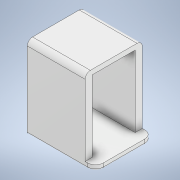
# Autodesk Inventor part: Fridge-Body
Saved by Autodesk Inventor 2020 (Build 240168000, 168)
## iProperties
Created: 2020-02-06
Part Number: Fridge-Body
Material: Generic
Document SubType Name: Modeling
Designer: Simon
Density: 1 g/cm^3
Appearance: Smooth - White
Author: Simon
Autodesk Inventor part; units mm, degrees
ref_plane "YZ Plane" through (0, 0, 0) normal (1, 0, 0) x (0, 1, 0)
ref_plane "XZ Plane" through (0, 0, 0) normal (0, 1, 0) x (-1, 0, 0)
ref_plane "XY Plane" through (0, 0, 0) normal (0, 0, 1) x (1, 0, 0)
sketch "Sketch1" plane through (0, 0, 0) normal (1, 0, 0) x (0, 1, 0)
  line L0 (0, 139.7) -> (396.875, 139.7)
  line L1 (396.875, 139.7) -> (396.875, -139.7)
  line L2 (396.875, -139.7) -> (0, -139.7)
  line L3 (0, -139.7) -> (0, 139.7)
  line L4 (396.875, -139.7) -> (0, 139.7) construction
  line L5 (23.8125, -104.775) -> (373.0625, -104.775)
  line L6 (373.0625, -104.775) -> (373.0625, 104.775)
  line L7 (373.0625, 104.775) -> (23.8125, 104.775)
  line L8 (23.8125, 104.775) -> (23.8125, -104.775)
  line L9 (23.8125, -104.775) -> (373.0625, 104.775) construction
  line L10 (373.0625, -104.775) -> (23.8125, 104.775) construction
  line L11 (23.8125, 104.775) -> (23.8125, 139.7)
  line L12 (23.8125, -104.775) -> (23.8125, -139.7)
  line L13 (198.4375, 104.775) -> (198.4375, -104.775)
  point P0 (0, 0)
  point P1 (0, 0)
  point P2 (198.4375, 0)
  dimension "d0" = 396.875
  dimension "d1" = 279.4
  dimension "d2" = 349.25
  dimension "d3" = 209.55
  constraints: 28 end point, 6 midpoint, 4 parallel, 3 perpendicular, 3 point on line, 2 horizontal, 1 coincident
  measures "d0" distance of L1.end L2.end
  measures "d1" distance of L0.end L1.end
  measures "d2" distance of L7.end L6.end
  measures "d3" distance of L6.end L5.end
extrude "Extrusion1" add sketch "Sketch1" against normal blind 282.575
extrude "Extrusion2" add sketch "Sketch1" along normal blind 50.8 contours L0 L11 L8 L12 L2 L3
extrude "Extrusion3" cut sketch "Sketch1" against normal blind 190.5 contours L7 L6 L5 L13
extrude "Extrusion4" cut sketch "Sketch1" against normal blind 247.65 contours L7 L13 L5 L8
fillet "Fillet3" radius 38.1 2 edges at (50.8, 11.9063, -139.7) (50.8, 11.9062, 139.7)
fillet "Fillet1" radius 25.4 2 edges at (-141.2875, 396.875, 139.7) (-141.2875, 396.875, -139.7)
fillet "Fillet2" radius 6.35 2 edges at (-134.9375, 0, 139.7) (-134.9375, 0, -139.7)
body "Solid1"
